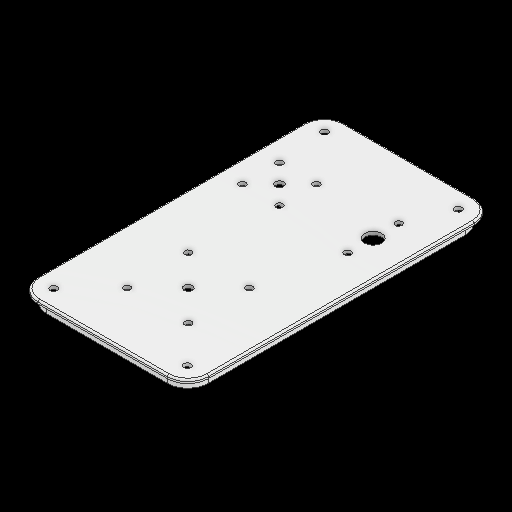
# Autodesk Inventor part: gora
Saved by Autodesk Inventor 2024.4 (Build 284460000, 460)
## iProperties
Created: 2026-02-13
Part Number: gora
Material: Tworzywo sztuczne ABS
Document SubType Name: Modeling
Designer: User
Density: 1.06 g/cm^3
Appearance: Gładki — biały
Author: User
Autodesk Inventor part; units mm, degrees
ref_plane "YZ Plane" through (0, 0, 0) normal (1, 0, 0) x (0, 1, 0)
ref_plane "XZ Plane" through (0, 0, 0) normal (0, 1, 0) x (-1, 0, 0)
ref_plane "XY Plane" through (0, 0, 0) normal (0, 0, 1) x (1, 0, 0)
sketch "Szkic1" plane through (0, 0, 0) normal (0, 1, 0) x (-1, 0, 0)
  line L0 (-47.5, 75.5) -> (-47.5, -75.5)
  line L1 (-35.5, -87.5) -> (35.5, -87.5)
  arc A0 (-47.5, -75.5) -> (-35.5, -87.5) centre (-35.5, -75.5) ccw
  line L2 (-50, 78) -> (-50, -78)
  line L3 (38, -90) -> (-38, -90)
  arc A1 (-50, -78) -> (-38, -90) centre (-38, -78) ccw
  arc A2 (35.5, -87.5) -> (47.5, -75.5) centre (35.5, -75.5) ccw
  line L4 (-35.5, -87.5) -> (35.5, -87.5)
  arc A3 (-50, -78) -> (-38, -90) centre (-38, -78) ccw
  line L5 (38, -90) -> (-38, -90)
  line L6 (-50, -78) -> (-50, 78)
  line L7 (-47.5, 75.5) -> (-47.5, -75.5)
  circle A4 centre (-39.2105, -79.5457) radius 2.6
  circle A5 centre (-39.2105, -79.5457) radius 2.6
  circle A6 centre (-39.2105, 79.5457) radius 2.6
  circle A7 centre (-39.2105, 79.5457) radius 2.6
  circle A8 centre (39.2105, 79.5457) radius 2.6
  circle A9 centre (39.2105, 79.5457) radius 2.6
  circle A10 centre (39.2105, -79.5457) radius 2.6
  circle A11 centre (39.2105, -79.5457) radius 2.6
  line L8 (50, -78) -> (50, 78)
  line L9 (50, -78) -> (50, 78)
  line L10 (38, 90) -> (-38, 90)
  line L11 (38, 90) -> (-38, 90)
  arc A12 (-35.5, 87.5) -> (-47.5, 75.5) centre (-35.5, 75.5) ccw
  arc A13 (47.5, 75.5) -> (35.5, 87.5) centre (35.5, 75.5) ccw
  line L12 (-35.5, 87.5) -> (35.5, 87.5)
  line L13 (47.5, 75.5) -> (47.5, -75.5)
  line L14 (47.5, 75.5) -> (47.5, -75.5)
  arc A14 (35.5, -87.5) -> (47.5, -75.5) centre (35.5, -75.5) ccw
  arc A15 (38, -90) -> (50, -78) centre (38, -78) ccw
  arc A16 (38, -90) -> (50, -78) centre (38, -78) ccw
  arc A17 (47.5, 75.5) -> (35.5, 87.5) centre (35.5, 75.5) ccw
  arc A18 (50, 78) -> (38, 90) centre (38, 78) ccw
  arc A19 (50, 78) -> (38, 90) centre (38, 78) ccw
  arc A20 (-38, 90) -> (-50, 78) centre (-38, 78) ccw
  arc A21 (-38, 90) -> (-50, 78) centre (-38, 78) ccw
  arc A22 (-35.5, 87.5) -> (-47.5, 75.5) centre (-35.5, 75.5) ccw
  line L15 (-46.55, 73.99) -> (-46.55, -73.99)
  line L16 (-34.79, -85.75) -> (34.79, -85.75)
  arc A23 (-46.55, -73.99) -> (-34.79, -85.75) centre (-34.79, -73.99) ccw
  arc A24 (34.79, -85.75) -> (46.55, -73.99) centre (34.79, -73.99) ccw
  line L17 (-34.79, -85.75) -> (34.79, -85.75)
  line L18 (-46.55, 73.99) -> (-46.55, -73.99)
  arc A25 (-34.79, 85.75) -> (-46.55, 73.99) centre (-34.79, 73.99) ccw
  arc A26 (46.55, 73.99) -> (34.79, 85.75) centre (34.79, 73.99) ccw
  line L19 (-34.79, 85.75) -> (34.79, 85.75)
  line L20 (46.55, 73.99) -> (46.55, -73.99)
  line L21 (46.55, 73.99) -> (46.55, -73.99)
  arc A27 (34.79, -85.75) -> (46.55, -73.99) centre (34.79, -73.99) ccw
  arc A28 (46.55, 73.99) -> (34.79, 85.75) centre (34.79, 73.99) ccw
  arc A29 (-34.79, 85.75) -> (-46.55, 73.99) centre (-34.79, 73.99) ccw
  point P0 (0, 0)
  point P1 (0, 0)
  point P2 (0, 0)
  constraints: 46 point on circle, 44 end point, 30 centre point, 18 tangent, 5 horizontal, 4 coincident, 2 collinear, 2 concentric, 2 vertical, 1 parallel
extrude "Wyciągnięcie proste1" add sketch "Szkic1" along normal blind 2 contours A12 L12 A13 L13 A2 L1 A0 L0 | A20 L10 A18 L8 A15 L3 A1 L2 | A4 | A6 | A8 | A10 | A25 L19 A26 L20 A24 L16 A23 L15
extrude "Wyciągnięcie proste2" add sketch "Szkic1" against normal blind 5 contours A12 L12 A13 L13 A2 L1 A0 L0
extrude "Wyciągnięcie proste3" cut sketch "Szkic1" along normal blind 5 contours A4 | A6 | A8 | A10
offset faces "Rozmiar3" outward -0.1 faces at (46.6705, -3.3333, -79.8841) (11.8333, -3.3333, -87.5) (47.5, -1.6667, 25.1667) (-45.8923, -3.3333, -81.5) (-47.5, -1.6667, -25.1667) (-43.6621, -3.3333, 84.2966) (-11.8333, -1.6667, 87.5) (47.366, -3.3333, 77.2885)
sketch "Szkic2" plane through (0, 0, 0) normal (0, -1, 0) x (1, 0, 0)
  line L0 (-46.6033, 85.9761) -> (46.6912, 85.9761) construction
  line L1 (46.6912, 85.9761) -> (46.6912, -85.8318) construction
  line L2 (46.6912, -85.8318) -> (-46.6033, -85.8318) construction
  line L3 (-46.6033, -85.8318) -> (-46.6033, 85.9761) construction
  line L4 (-21.1651, 35.5677) -> (-24.1992, 23.5677)
  line L5 (-24.1992, 23.5677) -> (-27.5055, 23.5677)
  line L6 (-27.5055, 23.5677) -> (-29.4309, 30.9875)
  line L7 (-29.4309, 30.9875) -> (-31.2883, 23.5677)
  line L8 (-31.2883, 23.5677) -> (-34.6044, 23.5677)
  line L9 (-34.6044, 23.5677) -> (-37.6384, 35.5677)
  line L10 (-37.6384, 35.5677) -> (-34.5071, 35.5677)
  line L11 (-34.5071, 35.5677) -> (-32.854, 27.5353)
  line L12 (-32.854, 27.5353) -> (-30.8507, 35.5677)
  line L13 (-30.8507, 35.5677) -> (-27.8556, 35.5677)
  line L14 (-27.8556, 35.5677) -> (-25.9496, 27.5256)
  line L15 (-25.9496, 27.5256) -> (-24.2186, 35.5677)
  line L16 (-24.2186, 35.5677) -> (-21.1651, 35.5677)
  spline S0 degree 2 poles (-15.204, 23.3246) (-17.7713, 23.3246) (-20.5039, 25.7752) (-20.5039, 28.041) knots 0 0 0 1 2 2 2
  spline S1 degree 2 poles (-20.5039, 28.041) (-20.5039, 30.2581) (-17.9561, 32.9032) (-15.6611, 32.9032) knots 0 0 0 1 2 2 2
  spline S2 degree 2 poles (-15.6611, 32.9032) (-13.5898, 32.9032) (-11.4893, 30.6568) (-11.4893, 28.5758) knots 0 0 0 1 2 2 2
  line L17 (-11.4893, 28.5758) -> (-11.4893, 27.5547)
  line L18 (-11.4893, 27.5547) -> (-17.6838, 27.5547)
  spline S3 degree 2 poles (-17.6838, 27.5547) (-17.6449, 26.9226) (-17.1878, 26.0863) (-16.8183, 25.8335) knots 0 0 0 1 2 2 2
  spline S4 degree 2 poles (-16.8183, 25.8335) (-16.4585, 25.5807) (-15.486, 25.3667) (-14.9123, 25.3667) knots 0 0 0 1 2 2 2
  spline S5 degree 2 poles (-14.9123, 25.3667) (-14.4261, 25.3667) (-13.4731, 25.5807) (-13.0744, 25.7654) knots 0 0 0 1 2 2 2
  spline S6 degree 2 poles (-13.0744, 25.7654) (-12.7243, 25.9113) (-12.1408, 26.2711) (-11.9561, 26.4073) knots 0 0 0 1 2 2 2
  line L19 (-11.9561, 26.4073) -> (-11.6546, 26.4073)
  line L20 (-11.6546, 26.4073) -> (-11.6546, 24.0734)
  spline S7 degree 2 poles (-11.6546, 24.0734) (-12.0047, 23.9372) (-12.5687, 23.7038) (-13.0744, 23.5872) knots 0 0 0 1 2 2 2
  spline S8 degree 2 poles (-13.0744, 23.5872) (-13.5314, 23.4607) (-14.5039, 23.3246) (-15.204, 23.3246) knots 0 0 0 1 2 2 2
  spline S9 degree 2 poles (-14.2705, 29.2565) (-14.2899, 30.1512) (-15.0776, 31.0944) (-15.8848, 31.0944) knots 0 0 0 1 2 2 2
  spline S10 degree 2 poles (-15.8848, 31.0944) (-16.7113, 31.0944) (-17.6449, 30.1026) (-17.6935, 29.2565) knots 0 0 0 1 2 2 2
  line L21 (-17.6935, 29.2565) -> (-14.2705, 29.2565)
  spline S11 degree 2 poles (-5.0517, 24.5304) (-5.3434, 24.2873) (-5.8005, 23.8983) (-6.1895, 23.7038) knots 0 0 0 1 2 2 2
  spline S12 degree 2 poles (-6.1895, 23.7038) (-6.5687, 23.5191) (-7.2883, 23.3246) (-7.9301, 23.3246) knots 0 0 0 1 2 2 2
  spline S13 degree 2 poles (-7.9301, 23.3246) (-9.136, 23.3246) (-10.7211, 24.9389) (-10.7211, 26.1641) knots 0 0 0 1 2 2 2
  spline S14 degree 2 poles (-10.7211, 26.1641) (-10.7211, 27.1658) (-9.9139, 28.4105) (-9.1554, 28.7703) knots 0 0 0 1 2 2 2
  spline S15 degree 2 poles (-9.1554, 28.7703) (-8.3872, 29.1398) (-6.2575, 29.4316) (-5.0322, 29.5094) knots 0 0 0 1 2 2 2
  line L22 (-5.0322, 29.5094) -> (-5.0322, 29.558)
  spline S16 degree 2 poles (-5.0322, 29.558) (-5.0322, 30.3068) (-6.1408, 30.8805) (-7.2494, 30.8805) knots 0 0 0 1 2 2 2
  spline S17 degree 2 poles (-7.2494, 30.8805) (-7.7454, 30.8805) (-9.0873, 30.5207) (-9.7194, 30.2387) knots 0 0 0 1 2 2 2
  line L23 (-9.7194, 30.2387) -> (-9.9625, 30.2387)
  line L24 (-9.9625, 30.2387) -> (-9.9625, 32.4267)
  spline S18 degree 2 poles (-9.9625, 32.4267) (-9.5444, 32.5434) (-7.6773, 32.874) (-6.7243, 32.874) knots 0 0 0 1 2 2 2
  spline S19 degree 2 poles (-6.7243, 32.874) (-4.3904, 32.874) (-2.251, 31.3181) (-2.251, 29.7233) knots 0 0 0 1 2 2 2
  line L25 (-2.251, 29.7233) -> (-2.251, 23.5677)
  line L26 (-2.251, 23.5677) -> (-5.0517, 23.5677)
  line L27 (-5.0517, 23.5677) -> (-5.0517, 24.5304)
  line L28 (-5.0517, 25.9308) -> (-5.0517, 27.8076)
  spline S20 degree 2 poles (-5.0517, 27.8076) (-5.7713, 27.7395) (-6.6562, 27.6325) (-7.0841, 27.4769) knots 0 0 0 1 2 2 2
  spline S21 degree 2 poles (-7.0841, 27.4769) (-7.4634, 27.3505) (-7.8718, 26.8254) (-7.8718, 26.3975) knots 0 0 0 1 2 2 2
  spline S22 degree 2 poles (-7.8718, 26.3975) (-7.8718, 25.7654) (-7.1813, 25.2889) (-6.5104, 25.2889) knots 0 0 0 1 2 2 2
  spline S23 degree 2 poles (-6.5104, 25.2889) (-6.1408, 25.2889) (-5.3629, 25.6293) (-5.0517, 25.9308) knots 0 0 0 1 2 2 2
  spline S24 degree 2 poles (3.3016, 23.3927) (1.5804, 23.3927) (0.005, 24.8124) (0.005, 26.4267) knots 0 0 0 1 2 2 2
  line L29 (0.005, 26.4267) -> (0.005, 30.6568)
  line L30 (0.005, 30.6568) -> (-1.0744, 30.6568)
  line L31 (-1.0744, 30.6568) -> (-1.0744, 32.6212)
  line L32 (-1.0744, 32.6212) -> (0.005, 32.6212)
  line L33 (0.005, 32.6212) -> (0.005, 35.2079)
  line L34 (0.005, 35.2079) -> (2.8251, 35.2079)
  line L35 (2.8251, 35.2079) -> (2.8251, 32.6212)
  line L36 (2.8251, 32.6212) -> (5.548, 32.6212)
  line L37 (5.548, 32.6212) -> (5.548, 30.6568)
  line L38 (5.548, 30.6568) -> (2.8251, 30.6568)
  line L39 (2.8251, 30.6568) -> (2.8251, 27.438)
  spline S25 degree 2 poles (2.8251, 27.438) (2.8251, 26.9615) (2.8446, 26.2517) (2.9613, 25.9697) knots 0 0 0 1 2 2 2
  spline S26 degree 2 poles (2.9613, 25.9697) (3.078, 25.6876) (3.6517, 25.357) (4.1963, 25.357) knots 0 0 0 1 2 2 2
  spline S27 degree 2 poles (4.1963, 25.357) (4.4297, 25.357) (5.159, 25.5515) (5.3049, 25.6293) knots 0 0 0 1 2 2 2
  line L40 (5.3049, 25.6293) -> (5.548, 25.6293)
  line L41 (5.548, 25.6293) -> (5.548, 23.6455)
  spline S28 degree 2 poles (5.548, 23.6455) (5.0909, 23.5288) (4.0601, 23.3927) (3.3016, 23.3927) knots 0 0 0 1 2 2 2
  line L42 (15.1655, 23.5677) -> (12.3259, 23.5677)
  line L43 (12.3259, 23.5677) -> (12.3259, 28.0507)
  spline S29 degree 2 poles (12.3259, 28.0507) (12.3259, 28.605) (12.2384, 29.6941) (12.1217, 29.947) knots 0 0 0 1 2 2 2
  spline S30 degree 2 poles (12.1217, 29.947) (11.9759, 30.2581) (11.4313, 30.5207) (10.9645, 30.5207) knots 0 0 0 1 2 2 2
  spline S31 degree 2 poles (10.9645, 30.5207) (10.6242, 30.5207) (9.9143, 30.2581) (9.5156, 29.9761) knots 0 0 0 1 2 2 2
  line L44 (9.5156, 29.9761) -> (9.5156, 23.5677)
  line L45 (9.5156, 23.5677) -> (6.6955, 23.5677)
  line L46 (6.6955, 23.5677) -> (6.6955, 36.1026)
  line L47 (6.6955, 36.1026) -> (9.5156, 36.1026)
  line L48 (9.5156, 36.1026) -> (9.5156, 31.6196)
  spline S32 degree 2 poles (9.5156, 31.6196) (10.206, 32.203) (11.5188, 32.8643) (12.3162, 32.8643) knots 0 0 0 1 2 2 2
  spline S33 degree 2 poles (12.3162, 32.8643) (13.6971, 32.8643) (15.1655, 31.1139) (15.1655, 29.4607) knots 0 0 0 1 2 2 2
  line L49 (15.1655, 29.4607) -> (15.1655, 23.5677)
  spline S34 degree 2 poles (21.8948, 23.3246) (19.3276, 23.3246) (16.595, 25.7752) (16.595, 28.041) knots 0 0 0 1 2 2 2
  spline S35 degree 2 poles (16.595, 28.041) (16.595, 30.2581) (19.1428, 32.9032) (21.4378, 32.9032) knots 0 0 0 1 2 2 2
  spline S36 degree 2 poles (21.4378, 32.9032) (23.5091, 32.9032) (25.6096, 30.6568) (25.6096, 28.5758) knots 0 0 0 1 2 2 2
  line L50 (25.6096, 28.5758) -> (25.6096, 27.5547)
  line L51 (25.6096, 27.5547) -> (19.4151, 27.5547)
  spline S37 degree 2 poles (19.4151, 27.5547) (19.454, 26.9226) (19.911, 26.0863) (20.2806, 25.8335) knots 0 0 0 1 2 2 2
  spline S38 degree 2 poles (20.2806, 25.8335) (20.6404, 25.5807) (21.6128, 25.3667) (22.1866, 25.3667) knots 0 0 0 1 2 2 2
  spline S39 degree 2 poles (22.1866, 25.3667) (22.6728, 25.3667) (23.6258, 25.5807) (24.0245, 25.7654) knots 0 0 0 1 2 2 2
  spline S40 degree 2 poles (24.0245, 25.7654) (24.3746, 25.9113) (24.958, 26.2711) (25.1428, 26.4073) knots 0 0 0 1 2 2 2
  line L52 (25.1428, 26.4073) -> (25.4443, 26.4073)
  line L53 (25.4443, 26.4073) -> (25.4443, 24.0734)
  spline S41 degree 2 poles (25.4443, 24.0734) (25.0942, 23.9372) (24.5302, 23.7038) (24.0245, 23.5872) knots 0 0 0 1 2 2 2
  spline S42 degree 2 poles (24.0245, 23.5872) (23.5674, 23.4607) (22.595, 23.3246) (21.8948, 23.3246) knots 0 0 0 1 2 2 2
  spline S43 degree 2 poles (22.8284, 29.2565) (22.8089, 30.1512) (22.0212, 31.0944) (21.2141, 31.0944) knots 0 0 0 1 2 2 2
  spline S44 degree 2 poles (21.2141, 31.0944) (20.3875, 31.0944) (19.454, 30.1026) (19.4054, 29.2565) knots 0 0 0 1 2 2 2
  line L54 (19.4054, 29.2565) -> (22.8284, 29.2565)
  line L55 (33.1363, 29.947) -> (32.9029, 29.947)
  spline S45 degree 2 poles (32.9029, 29.947) (32.7376, 30.0053) (32.125, 30.0637) (31.7554, 30.0637) knots 0 0 0 1 2 2 2
  spline S46 degree 2 poles (31.7554, 30.0637) (31.3178, 30.0637) (30.3357, 29.8011) (29.8786, 29.6261) knots 0 0 0 1 2 2 2
  line L56 (29.8786, 29.6261) -> (29.8786, 23.5677)
  line L57 (29.8786, 23.5677) -> (27.0585, 23.5677)
  line L58 (27.0585, 23.5677) -> (27.0585, 32.6212)
  line L59 (27.0585, 32.6212) -> (29.8786, 32.6212)
  line L60 (29.8786, 32.6212) -> (29.8786, 31.3181)
  spline S47 degree 2 poles (29.8786, 31.3181) (30.0731, 31.4932) (30.7538, 32.0377) (31.0358, 32.203) knots 0 0 0 1 2 2 2
  spline S48 degree 2 poles (31.0358, 32.203) (31.347, 32.3878) (32.1639, 32.6504) (32.5237, 32.6504) knots 0 0 0 1 2 2 2
  spline S49 degree 2 poles (32.5237, 32.6504) (32.6598, 32.6504) (33.0002, 32.6309) (33.1363, 32.6212) knots 0 0 0 1 2 2 2
  line L61 (33.1363, 32.6212) -> (33.1363, 29.947)
  spline S50 degree 2 poles (-27.3061, 3.5961) (-28.687, 3.5961) (-30.7681, 4.1309) (-31.6627, 4.5199) knots 0 0 0 1 2 2 2
  line L62 (-31.6627, 4.5199) -> (-31.6627, 7.3789)
  line L63 (-31.6627, 7.3789) -> (-31.3904, 7.3789)
  spline S51 degree 2 poles (-31.3904, 7.3789) (-30.4861, 6.6107) (-28.3175, 5.7841) (-27.2964, 5.7841) knots 0 0 0 1 2 2 2
  spline S52 degree 2 poles (-27.2964, 5.7841) (-27.0339, 5.7841) (-26.1878, 5.9008) (-25.935, 6.0175) knots 0 0 0 1 2 2 2
  spline S53 degree 2 poles (-25.935, 6.0175) (-25.6238, 6.1536) (-25.1862, 6.6496) (-25.1862, 7.0483) knots 0 0 0 1 2 2 2
  spline S54 degree 2 poles (-25.1862, 7.0483) (-25.1862, 7.5053) (-25.8961, 8.0693) (-26.3823, 8.1958) knots 0 0 0 1 2 2 2
  spline S55 degree 2 poles (-26.3823, 8.1958) (-26.995, 8.3611) (-28.3856, 8.6431) (-28.9982, 8.857) knots 0 0 0 1 2 2 2
  spline S56 degree 2 poles (-28.9982, 8.857) (-30.3888, 9.3432) (-31.5946, 11.0061) (-31.5946, 12.2509) knots 0 0 0 1 2 2 2
  spline S57 degree 2 poles (-31.5946, 12.2509) (-31.5946, 13.9332) (-28.7454, 16.024) (-26.606, 16.024) knots 0 0 0 1 2 2 2
  spline S58 degree 2 poles (-26.606, 16.024) (-25.5363, 16.024) (-23.4164, 15.5864) (-22.5801, 15.2168) knots 0 0 0 1 2 2 2
  line L64 (-22.5801, 15.2168) -> (-22.5801, 12.4745)
  line L65 (-22.5801, 12.4745) -> (-22.8426, 12.4745)
  spline S59 degree 2 poles (-22.8426, 12.4745) (-23.5136, 13.0483) (-25.439, 13.836) (-26.4504, 13.836) knots 0 0 0 1 2 2 2
  spline S60 degree 2 poles (-26.4504, 13.836) (-26.8491, 13.836) (-27.4715, 13.7193) (-27.8215, 13.5637) knots 0 0 0 1 2 2 2
  spline S61 degree 2 poles (-27.8215, 13.5637) (-28.1036, 13.4373) (-28.512, 12.9316) (-28.512, 12.6204) knots 0 0 0 1 2 2 2
  spline S62 degree 2 poles (-28.512, 12.6204) (-28.512, 12.1536) (-27.8604, 11.6188) (-26.9269, 11.4048) knots 0 0 0 1 2 2 2
  spline S63 degree 2 poles (-26.9269, 11.4048) (-26.324, 11.2687) (-25.2057, 11.0061) (-24.5638, 10.7825) knots 0 0 0 1 2 2 2
  spline S64 degree 2 poles (-24.5638, 10.7825) (-23.3191, 10.3254) (-22.1036, 8.8084) (-22.1036, 7.5637) knots 0 0 0 1 2 2 2
  spline S65 degree 2 poles (-22.1036, 7.5637) (-22.1036, 5.7744) (-24.9139, 3.5961) (-27.3061, 3.5961) knots 0 0 0 1 2 2 2
  spline S66 degree 2 poles (-17.2608, 3.635) (-18.982, 3.635) (-20.5574, 5.0548) (-20.5574, 6.669) knots 0 0 0 1 2 2 2
  line L66 (-20.5574, 6.669) -> (-20.5574, 10.8992)
  line L67 (-20.5574, 10.8992) -> (-21.6368, 10.8992)
  line L68 (-21.6368, 10.8992) -> (-21.6368, 12.8635)
  line L69 (-21.6368, 12.8635) -> (-20.5574, 12.8635)
  line L70 (-20.5574, 12.8635) -> (-20.5574, 15.4502)
  line L71 (-20.5574, 15.4502) -> (-17.7373, 15.4502)
  line L72 (-17.7373, 15.4502) -> (-17.7373, 12.8635)
  line L73 (-17.7373, 12.8635) -> (-15.0144, 12.8635)
  line L74 (-15.0144, 12.8635) -> (-15.0144, 10.8992)
  line L75 (-15.0144, 10.8992) -> (-17.7373, 10.8992)
  line L76 (-17.7373, 10.8992) -> (-17.7373, 7.6804)
  spline S67 degree 2 poles (-17.7373, 7.6804) (-17.7373, 7.2039) (-17.7178, 6.494) (-17.6011, 6.212) knots 0 0 0 1 2 2 2
  spline S68 degree 2 poles (-17.6011, 6.212) (-17.4844, 5.93) (-16.9107, 5.5993) (-16.3661, 5.5993) knots 0 0 0 1 2 2 2
  spline S69 degree 2 poles (-16.3661, 5.5993) (-16.1327, 5.5993) (-15.4034, 5.7938) (-15.2575, 5.8716) knots 0 0 0 1 2 2 2
  line L77 (-15.2575, 5.8716) -> (-15.0144, 5.8716)
  line L78 (-15.0144, 5.8716) -> (-15.0144, 3.8878)
  spline S70 degree 2 poles (-15.0144, 3.8878) (-15.4715, 3.7711) (-16.5023, 3.635) (-17.2608, 3.635) knots 0 0 0 1 2 2 2
  spline S71 degree 2 poles (-8.8783, 4.7727) (-9.17, 4.5296) (-9.6271, 4.1407) (-10.016, 3.9462) knots 0 0 0 1 2 2 2
  spline S72 degree 2 poles (-10.016, 3.9462) (-10.3953, 3.7614) (-11.1149, 3.5669) (-11.7567, 3.5669) knots 0 0 0 1 2 2 2
  spline S73 degree 2 poles (-11.7567, 3.5669) (-12.9625, 3.5669) (-14.5476, 5.1812) (-14.5476, 6.4065) knots 0 0 0 1 2 2 2
  spline S74 degree 2 poles (-14.5476, 6.4065) (-14.5476, 7.4081) (-13.7405, 8.6528) (-12.982, 9.0126) knots 0 0 0 1 2 2 2
  spline S75 degree 2 poles (-12.982, 9.0126) (-12.2138, 9.3821) (-10.0841, 9.6739) (-8.8588, 9.7517) knots 0 0 0 1 2 2 2
  line L79 (-8.8588, 9.7517) -> (-8.8588, 9.8003)
  spline S76 degree 2 poles (-8.8588, 9.8003) (-8.8588, 10.5491) (-9.9674, 11.1228) (-11.076, 11.1228) knots 0 0 0 1 2 2 2
  spline S77 degree 2 poles (-11.076, 11.1228) (-11.5719, 11.1228) (-12.9139, 10.763) (-13.546, 10.481) knots 0 0 0 1 2 2 2
  line L80 (-13.546, 10.481) -> (-13.7891, 10.481)
  line L81 (-13.7891, 10.481) -> (-13.7891, 12.669)
  spline S78 degree 2 poles (-13.7891, 12.669) (-13.371, 12.7857) (-11.5039, 13.1163) (-10.5509, 13.1163) knots 0 0 0 1 2 2 2
  spline S79 degree 2 poles (-10.5509, 13.1163) (-8.217, 13.1163) (-6.0776, 11.5604) (-6.0776, 9.9656) knots 0 0 0 1 2 2 2
  line L82 (-6.0776, 9.9656) -> (-6.0776, 3.81)
  line L83 (-6.0776, 3.81) -> (-8.8783, 3.81)
  line L84 (-8.8783, 3.81) -> (-8.8783, 4.7727)
  line L85 (-8.8783, 6.1731) -> (-8.8783, 8.0499)
  spline S80 degree 2 poles (-8.8783, 8.0499) (-9.5979, 7.9818) (-10.4828, 7.8749) (-10.9107, 7.7193) knots 0 0 0 1 2 2 2
  spline S81 degree 2 poles (-10.9107, 7.7193) (-11.2899, 7.5928) (-11.6984, 7.0677) (-11.6984, 6.6398) knots 0 0 0 1 2 2 2
  spline S82 degree 2 poles (-11.6984, 6.6398) (-11.6984, 6.0078) (-11.0079, 5.5313) (-10.3369, 5.5313) knots 0 0 0 1 2 2 2
  spline S83 degree 2 poles (-10.3369, 5.5313) (-9.9674, 5.5313) (-9.1895, 5.8716) (-8.8783, 6.1731) knots 0 0 0 1 2 2 2
  spline S84 degree 2 poles (-0.5249, 3.635) (-2.2462, 3.635) (-3.8215, 5.0548) (-3.8215, 6.669) knots 0 0 0 1 2 2 2
  line L86 (-3.8215, 6.669) -> (-3.8215, 10.8992)
  line L87 (-3.8215, 10.8992) -> (-4.901, 10.8992)
  line L88 (-4.901, 10.8992) -> (-4.901, 12.8635)
  line L89 (-4.901, 12.8635) -> (-3.8215, 12.8635)
  line L90 (-3.8215, 12.8635) -> (-3.8215, 15.4502)
  line L91 (-3.8215, 15.4502) -> (-1.0014, 15.4502)
  line L92 (-1.0014, 15.4502) -> (-1.0014, 12.8635)
  line L93 (-1.0014, 12.8635) -> (1.7214, 12.8635)
  line L94 (1.7214, 12.8635) -> (1.7214, 10.8992)
  line L95 (1.7214, 10.8992) -> (-1.0014, 10.8992)
  line L96 (-1.0014, 10.8992) -> (-1.0014, 7.6804)
  spline S85 degree 2 poles (-1.0014, 7.6804) (-1.0014, 7.2039) (-0.982, 6.494) (-0.8653, 6.212) knots 0 0 0 1 2 2 2
  spline S86 degree 2 poles (-0.8653, 6.212) (-0.7486, 5.93) (-0.1749, 5.5993) (0.3697, 5.5993) knots 0 0 0 1 2 2 2
  spline S87 degree 2 poles (0.3697, 5.5993) (0.6031, 5.5993) (1.3324, 5.7938) (1.4783, 5.8716) knots 0 0 0 1 2 2 2
  line L97 (1.4783, 5.8716) -> (1.7214, 5.8716)
  line L98 (1.7214, 5.8716) -> (1.7214, 3.8878)
  spline S88 degree 2 poles (1.7214, 3.8878) (1.2644, 3.7711) (0.2336, 3.635) (-0.5249, 3.635) knots 0 0 0 1 2 2 2
  line L99 (5.689, 3.81) -> (2.8689, 3.81)
  line L100 (2.8689, 3.81) -> (2.8689, 12.8635)
  line L101 (2.8689, 12.8635) -> (5.689, 12.8635)
  line L102 (5.689, 12.8635) -> (5.689, 3.81)
  line L103 (5.7765, 14.1569) -> (2.7911, 14.1569)
  line L104 (2.7911, 14.1569) -> (2.7911, 16.3546)
  line L105 (2.7911, 16.3546) -> (5.7765, 16.3546)
  line L106 (5.7765, 16.3546) -> (5.7765, 14.1569)
  spline S89 degree 2 poles (16.5318, 8.3319) (16.5318, 6.0953) (14.0909, 3.528) (11.864, 3.528) knots 0 0 0 1 2 2 2
  spline S90 degree 2 poles (11.864, 3.528) (9.6469, 3.528) (7.1866, 6.0953) (7.1866, 8.3319) knots 0 0 0 1 2 2 2
  spline S91 degree 2 poles (7.1866, 8.3319) (7.1866, 10.588) (9.6469, 13.1455) (11.864, 13.1455) knots 0 0 0 1 2 2 2
  spline S92 degree 2 poles (11.864, 13.1455) (14.0812, 13.1455) (16.5318, 10.5783) (16.5318, 8.3319) knots 0 0 0 1 2 2 2
  spline S93 degree 2 poles (13.6436, 8.3125) (13.6436, 9.1196) (13.3811, 10.199) (13.1477, 10.5199) knots 0 0 0 1 2 2 2
  spline S94 degree 2 poles (13.1477, 10.5199) (12.8948, 10.8603) (12.2627, 11.1228) (11.864, 11.1228) knots 0 0 0 1 2 2 2
  spline S95 degree 2 poles (11.864, 11.1228) (11.4751, 11.1228) (10.8624, 10.8894) (10.6096, 10.5588) knots 0 0 0 1 2 2 2
  spline S96 degree 2 poles (10.6096, 10.5588) (10.3665, 10.2476) (10.0747, 9.1488) (10.0747, 8.3125) knots 0 0 0 1 2 2 2
  spline S97 degree 2 poles (10.0747, 8.3125) (10.0747, 7.4859) (10.347, 6.4648) (10.5707, 6.1536) knots 0 0 0 1 2 2 2
  spline S98 degree 2 poles (10.5707, 6.1536) (10.7943, 5.8424) (11.4751, 5.5507) (11.8835, 5.5507) knots 0 0 0 1 2 2 2
  spline S99 degree 2 poles (11.8835, 5.5507) (12.2238, 5.5507) (12.924, 5.8424) (13.1379, 6.1342) knots 0 0 0 1 2 2 2
  spline S100 degree 2 poles (13.1379, 6.1342) (13.3811, 6.4745) (13.6436, 7.4567) (13.6436, 8.3125) knots 0 0 0 1 2 2 2
  line L107 (26.4994, 3.81) -> (23.6598, 3.81)
  line L108 (23.6598, 3.81) -> (23.6598, 8.293)
  spline S101 degree 2 poles (23.6598, 8.293) (23.6598, 8.8473) (23.5723, 9.9364) (23.4556, 10.1893) knots 0 0 0 1 2 2 2
  spline S102 degree 2 poles (23.4556, 10.1893) (23.3097, 10.5005) (22.7652, 10.763) (22.2984, 10.763) knots 0 0 0 1 2 2 2
  spline S103 degree 2 poles (22.2984, 10.763) (21.958, 10.763) (21.2481, 10.5005) (20.8494, 10.2184) knots 0 0 0 1 2 2 2
  line L109 (20.8494, 10.2184) -> (20.8494, 3.81)
  line L110 (20.8494, 3.81) -> (18.0293, 3.81)
  line L111 (18.0293, 3.81) -> (18.0293, 12.8635)
  line L112 (18.0293, 12.8635) -> (20.8494, 12.8635)
  line L113 (20.8494, 12.8635) -> (20.8494, 11.8619)
  spline S104 degree 2 poles (20.8494, 11.8619) (21.5399, 12.4454) (22.8527, 13.1066) (23.6501, 13.1066) knots 0 0 0 1 2 2 2
  spline S105 degree 2 poles (23.6501, 13.1066) (25.031, 13.1066) (26.4994, 11.3562) (26.4994, 9.7031) knots 0 0 0 1 2 2 2
  line L114 (26.4994, 9.7031) -> (26.4994, 3.81)
  line L115 (-26.8248, -35.7053) -> (-35.6449, -35.7053)
  line L116 (-35.6449, -35.7053) -> (-35.6449, -33.7507)
  spline S106 degree 2 poles (-35.6449, -33.7507) (-34.5266, -32.8561) (-32.7373, -31.2807) (-32.0663, -30.5708) knots 0 0 0 1 2 2 2
  spline S107 degree 2 poles (-32.0663, -30.5708) (-31.1813, -29.647) (-30.3937, -28.237) (-30.3937, -27.4979) knots 0 0 0 1 2 2 2
  spline S108 degree 2 poles (-30.3937, -27.4979) (-30.3937, -26.6616) (-31.3953, -25.7669) (-32.2899, -25.7669) knots 0 0 0 1 2 2 2
  spline S109 degree 2 poles (-32.2899, -25.7669) (-32.747, -25.7669) (-33.5638, -25.9906) (-33.982, -26.1656) knots 0 0 0 1 2 2 2
  spline S110 degree 2 poles (-33.982, -26.1656) (-34.3904, -26.3504) (-34.9739, -26.7394) (-35.1198, -26.8366) knots 0 0 0 1 2 2 2
  line L117 (-35.1198, -26.8366) -> (-35.3531, -26.8366)
  line L118 (-35.3531, -26.8366) -> (-35.3531, -24.2207)
  spline S111 degree 2 poles (-35.3531, -24.2207) (-34.8475, -23.9776) (-32.6886, -23.472) (-31.687, -23.472) knots 0 0 0 1 2 2 2
  spline S112 degree 2 poles (-31.687, -23.472) (-29.5476, -23.472) (-27.3499, -25.378) (-27.3499, -27.0992) knots 0 0 0 1 2 2 2
  spline S113 degree 2 poles (-27.3499, -27.0992) (-27.3499, -28.1592) (-28.3515, -30.2013) (-29.5087, -31.3682) knots 0 0 0 1 2 2 2
  spline S114 degree 2 poles (-29.5087, -31.3682) (-30.2381, -32.0878) (-31.6092, -33.2062) (-31.9107, -33.4395) knots 0 0 0 1 2 2 2
  line L119 (-31.9107, -33.4395) -> (-26.8248, -33.4395)
  line L120 (-26.8248, -33.4395) -> (-26.8248, -35.7053)
  spline S115 degree 2 poles (-16.4682, -29.7053) (-16.4682, -31.2613) (-16.9642, -33.5951) (-17.5185, -34.3828) knots 0 0 0 1 2 2 2
  spline S116 degree 2 poles (-17.5185, -34.3828) (-18.063, -35.1608) (-19.8232, -35.9582) (-21.0873, -35.9582) knots 0 0 0 1 2 2 2
  spline S117 degree 2 poles (-21.0873, -35.9582) (-22.3613, -35.9582) (-24.1117, -35.1608) (-24.666, -34.3634) knots 0 0 0 1 2 2 2
  spline S118 degree 2 poles (-24.666, -34.3634) (-25.2202, -33.5757) (-25.7162, -31.2613) (-25.7162, -29.7053) knots 0 0 0 1 2 2 2
  spline S119 degree 2 poles (-25.7162, -29.7053) (-25.7162, -28.1105) (-25.2202, -25.8545) (-24.6562, -25.0376) knots 0 0 0 1 2 2 2
  spline S120 degree 2 poles (-24.6562, -25.0376) (-24.0922, -24.2402) (-22.3126, -23.4622) (-21.0873, -23.4622) knots 0 0 0 1 2 2 2
  spline S121 degree 2 poles (-21.0873, -23.4622) (-19.794, -23.4622) (-18.063, -24.2791) (-17.5087, -25.0862) knots 0 0 0 1 2 2 2
  spline S122 degree 2 poles (-17.5087, -25.0862) (-16.9642, -25.8739) (-16.4682, -28.1981) (-16.4682, -29.7053) knots 0 0 0 1 2 2 2
  spline S123 degree 2 poles (-19.4925, -29.7053) (-19.4925, -27.4784) (-20.2219, -25.6794) (-21.0873, -25.6794) knots 0 0 0 1 2 2 2
  spline S124 degree 2 poles (-21.0873, -25.6794) (-21.9528, -25.6794) (-22.6919, -27.4784) (-22.6919, -29.7151) knots 0 0 0 1 2 2 2
  spline S125 degree 2 poles (-22.6919, -29.7151) (-22.6919, -31.9128) (-21.9528, -33.741) (-21.0873, -33.741) knots 0 0 0 1 2 2 2
  spline S126 degree 2 poles (-21.0873, -33.741) (-20.2316, -33.741) (-19.4925, -31.9128) (-19.4925, -29.7053) knots 0 0 0 1 2 2 2
  line L121 (-5.8005, -35.7053) -> (-14.6206, -35.7053)
  line L122 (-14.6206, -35.7053) -> (-14.6206, -33.7507)
  spline S127 degree 2 poles (-14.6206, -33.7507) (-13.5023, -32.8561) (-11.713, -31.2807) (-11.042, -30.5708) knots 0 0 0 1 2 2 2
  spline S128 degree 2 poles (-11.042, -30.5708) (-10.157, -29.647) (-9.3694, -28.237) (-9.3694, -27.4979) knots 0 0 0 1 2 2 2
  spline S129 degree 2 poles (-9.3694, -27.4979) (-9.3694, -26.6616) (-10.371, -25.7669) (-11.2656, -25.7669) knots 0 0 0 1 2 2 2
  spline S130 degree 2 poles (-11.2656, -25.7669) (-11.7227, -25.7669) (-12.5395, -25.9906) (-12.9577, -26.1656) knots 0 0 0 1 2 2 2
  spline S131 degree 2 poles (-12.9577, -26.1656) (-13.3661, -26.3504) (-13.9496, -26.7394) (-14.0954, -26.8366) knots 0 0 0 1 2 2 2
  line L123 (-14.0954, -26.8366) -> (-14.3288, -26.8366)
  line L124 (-14.3288, -26.8366) -> (-14.3288, -24.2207)
  spline S132 degree 2 poles (-14.3288, -24.2207) (-13.8232, -23.9776) (-11.6643, -23.472) (-10.6627, -23.472) knots 0 0 0 1 2 2 2
  spline S133 degree 2 poles (-10.6627, -23.472) (-8.5233, -23.472) (-6.3256, -25.378) (-6.3256, -27.0992) knots 0 0 0 1 2 2 2
  spline S134 degree 2 poles (-6.3256, -27.0992) (-6.3256, -28.1592) (-7.3272, -30.2013) (-8.4844, -31.3682) knots 0 0 0 1 2 2 2
  spline S135 degree 2 poles (-8.4844, -31.3682) (-9.2138, -32.0878) (-10.5849, -33.2062) (-10.8864, -33.4395) knots 0 0 0 1 2 2 2
  line L125 (-10.8864, -33.4395) -> (-5.8005, -33.4395)
  line L126 (-5.8005, -33.4395) -> (-5.8005, -35.7053)
  spline S136 degree 2 poles (4.6436, -31.6211) (4.6436, -33.5173) (2.2417, -35.9582) (0.1412, -35.9582) knots 0 0 0 1 2 2 2
  spline S137 degree 2 poles (0.1412, -35.9582) (-0.9091, -35.9582) (-2.5525, -35.3553) (-3.1262, -34.7621) knots 0 0 0 1 2 2 2
  spline S138 degree 2 poles (-3.1262, -34.7621) (-3.807, -34.0716) (-4.5363, -31.8836) (-4.5363, -30.3569) knots 0 0 0 1 2 2 2
  spline S139 degree 2 poles (-4.5363, -30.3569) (-4.5363, -28.7815) (-3.8556, -26.331) (-3.0873, -25.3877) knots 0 0 0 1 2 2 2
  spline S140 degree 2 poles (-3.0873, -25.3877) (-2.358, -24.493) (0.0148, -23.4817) (1.6387, -23.4817) knots 0 0 0 1 2 2 2
  spline S141 degree 2 poles (1.6387, -23.4817) (2.2319, -23.4817) (3.4183, -23.6373) (3.6323, -23.6859) knots 0 0 0 1 2 2 2
  line L127 (3.6323, -23.6859) -> (3.6323, -26.0392)
  line L128 (3.6323, -26.0392) -> (3.4183, -26.0392)
  spline S142 degree 2 poles (3.4183, -26.0392) (3.2044, -25.9323) (2.2319, -25.6697) (1.6096, -25.6697) knots 0 0 0 1 2 2 2
  spline S143 degree 2 poles (1.6096, -25.6697) (0.1995, -25.6697) (-1.3369, -27.1575) (-1.5217, -28.5384) knots 0 0 0 1 2 2 2
  spline S144 degree 2 poles (-1.5217, -28.5384) (-0.9285, -28.1592) (0.287, -27.7118) (1.0553, -27.7118) knots 0 0 0 1 2 2 2
  spline S145 degree 2 poles (1.0553, -27.7118) (1.7068, -27.7118) (2.8446, -28.0619) (3.2822, -28.3925) knots 0 0 0 1 2 2 2
  spline S146 degree 2 poles (3.2822, -28.3925) (3.9046, -28.869) (4.6436, -30.4152) (4.6436, -31.6211) knots 0 0 0 1 2 2 2
  spline S147 degree 2 poles (1.1331, -33.4298) (1.3665, -33.1381) (1.6193, -32.4574) (1.6193, -31.7669) knots 0 0 0 1 2 2 2
  spline S148 degree 2 poles (1.6193, -31.7669) (1.6193, -31.1835) (1.3276, -30.425) (1.065, -30.2013) knots 0 0 0 1 2 2 2
  spline S149 degree 2 poles (1.065, -30.2013) (0.7927, -29.9679) (0.1217, -29.8026) (-0.2575, -29.8026) knots 0 0 0 1 2 2 2
  spline S150 degree 2 poles (-0.2575, -29.8026) (-0.5784, -29.8026) (-1.2397, -29.9679) (-1.5314, -30.0846) knots 0 0 0 1 2 2 2
  spline S151 degree 2 poles (-1.5314, -30.0846) (-1.5314, -30.1624) (-1.5509, -30.5319) (-1.5509, -30.8139) knots 0 0 0 1 2 2 2
  spline S152 degree 2 poles (-1.5509, -30.8139) (-1.5509, -31.8545) (-1.1911, -33.1089) (-0.9091, -33.4298) knots 0 0 0 1 2 2 2
  spline S153 degree 2 poles (-0.9091, -33.4298) (-0.7048, -33.6924) (-0.1603, -33.916) (0.1315, -33.916) knots 0 0 0 1 2 2 2
  spline S154 degree 2 poles (0.1315, -33.916) (0.3746, -33.916) (0.9386, -33.6729) (1.1331, -33.4298) knots 0 0 0 1 2 2 2
  spline S155 degree 2 poles (20.8543, -32.0295) (20.8543, -32.9241) (20.1736, -34.2759) (19.6096, -34.7232) knots 0 0 0 1 2 2 2
  spline S156 degree 2 poles (19.6096, -34.7232) (18.9289, -35.258) (17.3146, -35.7053) (16.0601, -35.7053) knots 0 0 0 1 2 2 2
  line L129 (16.0601, -35.7053) -> (11.266, -35.7053)
  line L130 (11.266, -35.7053) -> (11.266, -23.7053)
  line L131 (11.266, -23.7053) -> (15.4961, -23.7053)
  spline S157 degree 2 poles (15.4961, -23.7053) (16.8187, -23.7053) (18.1801, -23.9096) (18.7733, -24.2305) knots 0 0 0 1 2 2 2
  spline S158 degree 2 poles (18.7733, -24.2305) (19.4248, -24.5708) (20.0569, -25.7378) (20.0569, -26.4963) knots 0 0 0 1 2 2 2
  spline S159 degree 2 poles (20.0569, -26.4963) (20.0569, -27.3715) (19.1817, -28.7426) (18.4037, -29.0635) knots 0 0 0 1 2 2 2
  line L132 (18.4037, -29.0635) -> (18.4037, -29.1219)
  spline S160 degree 2 poles (18.4037, -29.1219) (19.5221, -29.3553) (20.8543, -30.8042) (20.8543, -32.0295) knots 0 0 0 1 2 2 2
  spline S161 degree 2 poles (17.7425, -31.9809) (17.7425, -31.4169) (17.2952, -30.7848) (16.8478, -30.6194) knots 0 0 0 1 2 2 2
  spline S162 degree 2 poles (16.8478, -30.6194) (16.5755, -30.5125) (15.6128, -30.493) (14.8154, -30.493) knots 0 0 0 1 2 2 2
  line L133 (14.8154, -30.493) -> (14.2611, -30.493)
  line L134 (14.2611, -30.493) -> (14.2611, -33.5173)
  line L135 (14.2611, -33.5173) -> (14.4264, -33.5173)
  spline S163 degree 2 poles (14.4264, -33.5173) (15.5934, -33.5173) (16.488, -33.4882) (16.9548, -33.284) knots 0 0 0 1 2 2 2
  spline S164 degree 2 poles (16.9548, -33.284) (17.3632, -33.0992) (17.7425, -32.4185) (17.7425, -31.9809) knots 0 0 0 1 2 2 2
  spline S165 degree 2 poles (16.9937, -27.0895) (16.9937, -26.7977) (16.6922, -26.1851) (16.3811, -26.0489) knots 0 0 0 1 2 2 2
  spline S166 degree 2 poles (16.3811, -26.0489) (16.0893, -25.9128) (15.2725, -25.8934) (14.4653, -25.8934) knots 0 0 0 1 2 2 2
  line L136 (14.4653, -25.8934) -> (14.2611, -25.8934)
  line L137 (14.2611, -25.8934) -> (14.2611, -28.4412)
  line L138 (14.2611, -28.4412) -> (14.6404, -28.4412)
  spline S167 degree 2 poles (14.6404, -28.4412) (15.4086, -28.4412) (16.031, -28.412) (16.3616, -28.2564) knots 0 0 0 1 2 2 2
  spline S168 degree 2 poles (16.3616, -28.2564) (16.7214, -28.0814) (16.9937, -27.4882) (16.9937, -27.0895) knots 0 0 0 1 2 2 2
  line L139 (25.3373, -35.7053) -> (22.488, -35.7053)
  line L140 (22.488, -35.7053) -> (22.488, -32.5352)
  line L141 (22.488, -32.5352) -> (25.3373, -32.5352)
  line L142 (25.3373, -32.5352) -> (25.3373, -35.7053)
  spline S169 degree 2 poles (31.4443, -35.9193) (30.0634, -35.9193) (27.9823, -35.3844) (27.0877, -34.9955) knots 0 0 0 1 2 2 2
  line L143 (27.0877, -34.9955) -> (27.0877, -32.1365)
  line L144 (27.0877, -32.1365) -> (27.36, -32.1365)
  spline S170 degree 2 poles (27.36, -32.1365) (28.2644, -32.9047) (30.4329, -33.7313) (31.454, -33.7313) knots 0 0 0 1 2 2 2
  spline S171 degree 2 poles (31.454, -33.7313) (31.7165, -33.7313) (32.5626, -33.6146) (32.8154, -33.4979) knots 0 0 0 1 2 2 2
  spline S172 degree 2 poles (32.8154, -33.4979) (33.1266, -33.3617) (33.5642, -32.8658) (33.5642, -32.4671) knots 0 0 0 1 2 2 2
  spline S173 degree 2 poles (33.5642, -32.4671) (33.5642, -32.01) (32.8543, -31.446) (32.3681, -31.3196) knots 0 0 0 1 2 2 2
  spline S174 degree 2 poles (32.3681, -31.3196) (31.7554, -31.1543) (30.3648, -30.8723) (29.7522, -30.6583) knots 0 0 0 1 2 2 2
  spline S175 degree 2 poles (29.7522, -30.6583) (28.3616, -30.1721) (27.1558, -28.5092) (27.1558, -27.2645) knots 0 0 0 1 2 2 2
  spline S176 degree 2 poles (27.1558, -27.2645) (27.1558, -25.5822) (30.005, -23.4914) (32.1444, -23.4914) knots 0 0 0 1 2 2 2
  spline S177 degree 2 poles (32.1444, -23.4914) (33.2141, -23.4914) (35.3341, -23.929) (36.1704, -24.2985) knots 0 0 0 1 2 2 2
  line L145 (36.1704, -24.2985) -> (36.1704, -27.0408)
  line L146 (36.1704, -27.0408) -> (35.9078, -27.0408)
  spline S178 degree 2 poles (35.9078, -27.0408) (35.2368, -26.4671) (33.3114, -25.6794) (32.3, -25.6794) knots 0 0 0 1 2 2 2
  spline S179 degree 2 poles (32.3, -25.6794) (31.9013, -25.6794) (31.2789, -25.7961) (30.9289, -25.9517) knots 0 0 0 1 2 2 2
  spline S180 degree 2 poles (30.9289, -25.9517) (30.6469, -26.0781) (30.2384, -26.5838) (30.2384, -26.895) knots 0 0 0 1 2 2 2
  spline S181 degree 2 poles (30.2384, -26.895) (30.2384, -27.3617) (30.89, -27.8966) (31.8235, -28.1105) knots 0 0 0 1 2 2 2
  spline S182 degree 2 poles (31.8235, -28.1105) (32.4264, -28.2467) (33.5447, -28.5092) (34.1866, -28.7329) knots 0 0 0 1 2 2 2
  spline S183 degree 2 poles (34.1866, -28.7329) (35.4313, -29.19) (36.6469, -30.707) (36.6469, -31.9517) knots 0 0 0 1 2 2 2
  spline S184 degree 2 poles (36.6469, -31.9517) (36.6469, -33.741) (33.8365, -35.9193) (31.4443, -35.9193) knots 0 0 0 1 2 2 2
  point P0 (0, 0)
  constraints: 2 other
extrude "Wyciągnięcie proste4" cut sketch "Szkic2" against normal blind 0.6
offset faces "Rozmiar4" outward 0.5 faces at (-41.8021, 0.6667, 79.7549) (36.619, 0.6667, 79.7549) (-41.8021, 0.6667, -79.3365) (36.619, 0.6667, -79.3365)
sketch "Szkic3" plane through (0, 2, 0) normal (0, 1, 0) x (1, 0, 0)
  circle A0 centre (-39.2105, -79.5457) radius 2.1 projected
  circle A1 centre (-39.2105, 79.5457) radius 2.1 projected
  line L0 (-39.2105, -79.5457) -> (-39.2105, 79.5457)
  circle A2 centre (39.2105, 79.5457) radius 2.1 projected
  line L1 (-39.2105, 79.5457) -> (39.2105, 79.5457)
  circle A3 centre (39.2105, -79.5457) radius 2.1 projected
  line L2 (39.2105, 79.5457) -> (39.2105, -79.5457)
  line L3 (39.2105, -79.5457) -> (-39.2105, -79.5457)
  line L4 (-39.2105, -79.5457) -> (-39.2105, 0)
  line L5 (0, 0) -> (-39.2105, 0)
  line L6 (0, 0) -> (0, -79.5457)
  line L7 (0, 0) -> (0, 79.5457)
  line L8 (0, 0) -> (39.2105, 0)
  line L9 (25, -64.7729) -> (-25, -64.7729)
  line L10 (-25, -64.7729) -> (-25, -14.7729)
  line L11 (-25, -14.7729) -> (25, -14.7729)
  line L12 (25, -14.7729) -> (25, -64.7729)
  line L13 (25, -64.7729) -> (-25, -14.7729) construction
  line L14 (-25, -64.7729) -> (25, -14.7729) construction
  line L15 (-25, -64.7729) -> (-17.9289, -57.7018)
  line L16 (-25, -39.7729) -> (25, -39.7729)
  line L17 (0, -64.7729) -> (0, -14.7729)
  circle A4 centre (-17.9289, -57.7018) radius 2
  circle A5 centre (-17.9289, -21.8439) radius 2
  circle A6 centre (17.9289, -57.7018) radius 2
  circle A7 centre (17.9289, -21.8439) radius 2
  circle A8 centre (0, -39.7729) radius 2.5
  line L18 (0, 0) -> (0, 79.5457)
  line L19 (25, 64.7729) -> (-25, 64.7729)
  line L20 (-25, 64.7729) -> (-25, 14.7729)
  line L21 (-25, 14.7729) -> (25, 14.7729)
  line L22 (25, 14.7729) -> (25, 64.7729)
  line L23 (25, 64.7729) -> (-25, 14.7729) construction
  line L24 (-25, 64.7729) -> (25, 14.7729) construction
  line L25 (-25, 64.7729) -> (-17.9289, 57.7018)
  line L26 (-25, 39.7729) -> (25, 39.7729)
  line L27 (0, 64.7729) -> (0, 14.7729)
  circle A9 centre (-17.9289, 57.7018) radius 2
  circle A10 centre (-17.9289, 21.8439) radius 2
  circle A11 centre (17.9289, 57.7018) radius 2
  circle A12 centre (17.9289, 21.8439) radius 2
  circle A13 centre (0, 39.7729) radius 2.5
  line L28 (-25, 14.7729) -> (-17.9289, 21.8439)
  circle A14 centre (-17.9289, 21.8439) radius 2
  line L29 (-25, 14.7729) -> (-10.8579, 28.915)
  circle A15 centre (-10.8579, 28.915) radius 2
  circle A16 centre (10.8579, 28.915) radius 2
  circle A17 centre (-10.8579, 50.6307) radius 2
  circle A18 centre (10.8579, 50.6307) radius 2
  line L30 (-10.8579, 28.915) -> (-36.8579, 28.915)
  line L31 (-10.8579, 50.6307) -> (-36.8579, 50.6307)
  line L32 (-10.8579, 50.6307) -> (15.1421, 50.6307) construction
  line L33 (10.8579, 50.6307) -> (-15.1421, 50.6307)
  line L34 (10.8579, 28.915) -> (-15.1421, 28.915)
  line L35 (10.8579, 28.915) -> (36.8579, 28.915) construction
  circle A19 centre (-36.8579, 28.915) radius 2
  circle A20 centre (-36.8579, 50.6307) radius 2
  circle A21 centre (-15.1421, 50.6307) radius 2
  circle A22 centre (-15.1421, 28.915) radius 2
  line L36 (-36.8579, 50.6307) -> (-15.1421, 28.915)
  circle A23 centre (-26, 39.7729) radius 2.5
  line L37 (-26, 39.7729) -> (29, 39.7729)
  circle A24 centre (29, 39.7729) radius 5
  line L38 (29, 39.7729) -> (29, 54.7729)
  line L39 (29, 39.7729) -> (29, 24.7729)
  circle A25 centre (29, 24.7729) radius 2
  circle A26 centre (29, 54.7729) radius 2
  dimension "d12" = 50
  dimension "d13" = 50
  dimension "d14" = 10
  dimension "d15" = 4
  dimension "d18" = 5
  dimension "d25" = 20
  dimension "d26" = 4
  dimension "d27" = 26
  dimension "d28" = 26
  dimension "d29" = 180
  dimension "d30" = 26
  dimension "d31" = 26
  dimension "d32" = 180
  dimension "d33" = 4
  dimension "d34" = 4
  dimension "d35" = 4
  dimension "d36" = 4
  dimension "d38" = 5
  dimension "d39" = 55
  dimension "d40" = 10
  dimension "d41" = 15
  dimension "d42" = 15
  dimension "d43" = 4
  dimension "d44" = 4
  constraints: 80 end point, 23 centre point, 21 symmetric about line, 13 coincident, 12 midpoint, 7 perpendicular, 6 horizontal, 4 point on line, 3 collinear, 2 parallel, 2 vertical, 1 concentric, 11 other
  measures "d12" distance of L10.end L11.end
  measures "d13" distance of L9.end L10.end
  measures "d14" distance of L9.end L15.end
  measures "d15" diameter of A4
  measures "d18" diameter of A8
  measures "d25" distance of L20.end L29.end
  measures "d26" diameter of A15
  measures "d27" distance of L30.start L30.end
  measures "d28" distance of L31.start L31.end
  measures "d29" angle of L31 L32
  measures "d30" distance of L33.start L33.end
  measures "d31" distance of L34.start L34.end
  measures "d32" angle of L34 L35
  measures "d33" diameter of A19
  measures "d34" diameter of A20
  measures "d35" diameter of A21
  measures "d36" diameter of A22
  measures "d38" diameter of A23
  measures "d39" distance of L37.start L37.end
  measures "d40" diameter of A24
  measures "d41" distance of L38.start L38.end
  measures "d42" distance of L38.start L39.end
  measures "d43" diameter of A25
  measures "d44" diameter of A26
extrude "Wyciągnięcie proste5" cut sketch "Szkic3" against normal blind 10 contours A8 L16 L6 | L6 L16 A8 | L16 A8 L6 | L6 A8 L16 | A24 L26 L22 | L22 L37 L39 A24 | A23 L36 L20 | L20 L36 A23 | A22 L36 L30 | L30 A22 | L26 A24 L22 | L22 A24 L38 L37 | L39 L38 A24 | A23 L36 L20 L26 | L26 L20 A23 | L30 L36 A22 | L36 L37 L20 | A23 L20 L37 L36 | A21 L31 | L31 A21 | A20 L36 L31 | L31 L36 A20 | A4 | A5 | A6 | A7 | A19 | A25 | A26
ref_plane "Płaszczyzna konstrukcyjna1" through (-35.5, 0, -2.6) normal (0, 0, 1) x (1, 0, 0)
fillet "Zaokrąglenie1" radius 1 8 edges at (46.4853, 2, -86.4853) (0, 2, -90) (-46.4853, 2, -86.4853) (-50, 2, 0) (-46.4853, 2, 86.4853) (0, 2, 90) (46.4853, 2, 86.4853) (50, 2, 0)
